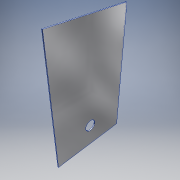
# Autodesk Inventor part: Inner Plate
Saved by Autodesk Inventor 2019 (Build 230136000, 136)
## iProperties
Created: 2018-10-04
Part Number: Inner Plate
Material: Aluminum 6061
Document SubType Name: Modeling
Designer: Adhik
Density: 2.7 g/cm^3
Appearance: Aluminum - Flat
Author: Adhik
Autodesk Inventor part; units mm, degrees
ref_plane "YZ Plane" through (0, 0, 0) normal (1, 0, 0) x (0, 1, 0)
ref_plane "XZ Plane" through (0, 0, 0) normal (0, 1, 0) x (-1, 0, 0)
ref_plane "XY Plane" through (0, 0, 0) normal (0, 0, 1) x (1, 0, 0)
sketch "Sketch1" plane through (0, 0, 0) normal (1, 0, 0) x (0, 1, 0)
  line L0 (0, -88.9) -> (0, 88.9) construction
  line L1 (-142.24, 0) -> (142.24, 0) construction
  line L2 (101.6, 63.5) -> (-101.6, 63.5)
  line L3 (-101.6, 63.5) -> (-101.6, -63.5)
  line L4 (-101.6, -63.5) -> (101.6, -63.5)
  line L5 (101.6, -63.5) -> (101.6, 63.5)
  circle A0 centre (-63.5, 0) radius 9.525
  circle A1 centre (-63.5, 0) radius 9.525 construction
  point P0 (0, 0)
  point P1 (101.6, 0)
  point P2 (0, 63.5)
  dimension "d0" = 203.2
  dimension "d1" = 127
  dimension "d3" = 19.05
  constraints: 8 end point, 3 point on line, 2 midpoint, 2 parallel, 1 centre point, 1 coincident, 1 horizontal, 1 perpendicular
  measures "d0" distance of L2.start L2.end
  measures "d1" distance of L4.end L2.start
  measures "d3" diameter of A0
extrude "Extrusion1" add sketch "Sketch1" along normal blind 1.5875
body "Solid1"
